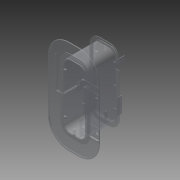
# Autodesk Inventor part: coil_former_lv_new
Saved by Autodesk Inventor 2014 SP1 (Build 180222100, 222)
## iProperties
Created: 2016-09-07
Part Number: coil_former_lv_new
Material: Polycarbonate, Clear
Document SubType Name: Modeling
Designer: tguillod
Density: 1.2 g/cm^3
Appearance: Polycarbonate - Clear
Author: tguillod
Autodesk Inventor part; units mm, degrees
ref_plane "YZ Plane" through (0, 0, 0) normal (1, 0, 0) x (0, 1, 0)
ref_plane "XZ Plane" through (0, 0, 0) normal (0, 1, 0) x (-1, 0, 0)
ref_plane "XY Plane" through (0, 0, 0) normal (0, 0, 1) x (1, 0, 0)
sketch "Sketch1" plane through (0, 0, 0) normal (0, 0, 1) x (1, 0, 0)
  line L0 (0, 0) -> (28, 0)
  line L1 (28, 0) -> (28, 1)
  line L2 (28, 1) -> (1, 1)
  line L3 (1, 1) -> (1, 3)
  line L4 (1, 3) -> (8, 3)
  line L5 (8, 3) -> (8, 4)
  line L6 (8, 4) -> (1, 4)
  line L7 (1, 4) -> (1, 55.5)
  line L8 (1, 55.5) -> (8, 55.5)
  line L9 (8, 55.5) -> (8, 56.5)
  line L10 (8, 56.5) -> (1, 56.5)
  line L11 (1, 56.5) -> (1, 59.5)
  line L12 (1, 59.5) -> (0, 59.5)
  line L13 (0, 59.5) -> (0, 0)
  line L14 (1, 58.5) -> (2, 58.5)
  line L15 (2, 58.5) -> (2, 57.5)
  line L16 (2, 57.5) -> (1, 57.5)
  line L17 (1, 57.5) -> (1, 58.5)
  line L18 (27, 1) -> (26, 1)
  line L19 (26, 1) -> (26, 2)
  line L20 (26, 2) -> (27, 2)
  line L21 (27, 2) -> (27, 1)
  dimension "d0" = 1
  dimension "d1" = 1
  dimension "d2" = 1
  dimension "d3" = 1
  dimension "d7" = 7
  dimension "d8" = 28
  dimension "d11" = 3
  dimension "d12" = 3
  dimension "d13" = 59.5
  dimension "d14" = 1
  dimension "d15" = 1
  dimension "d16" = 1
  dimension "d17" = 1
  dimension "d18" = 1
  dimension "d19" = 1
  dimension "d25" = 51.5
  constraints: 44 end point, 16 parallel, 3 collinear, 3 horizontal, 3 perpendicular, 2 point on line
  measures "d0" distance of L0.end L1.end
  measures "d1" distance of L4.end L5.end
  measures "d2" distance of L8.end L9.end
  measures "d3" distance of L11.end L12.end
  measures "d7" distance of L7.end L8.end
  measures "d8" distance of L0.start L0.end
  measures "d11" distance between parallel lines of L10 L12
  measures "d12" distance between parallel lines of L4 L0
  measures "d13" distance of L12.end L0.start
  measures "d14" distance of L18.end L19.end
  measures "d15" distance between parallel lines of L1 L21
  measures "d16" distance of L19.end L20.end
  measures "d17" distance of L15.end L16.end
  measures "d18" distance of L14.end L15.end
  measures "d19" distance between parallel lines of L12 L14
  measures "d25" distance between parallel lines of L6 L8
sketch "Sketch2" plane through (0, 0, 0) normal (0, 1, 0) x (-1, 0, 0)
  line L0 (0, 0) -> (0, 46.75)
  line L1 (10, 56.75) -> (18.5, 56.75)
  arc A0 (10, 56.75) -> (0, 46.75) centre (10, 46.75) ccw
  point P0 (0, 56.75)
  dimension "d20" = 56.75
  dimension "d21" = 18.5
  dimension "d22" = 10
  constraints: 4 end point, 2 point on circle, 2 point on line, 2 tangent, 1 centre point, 1 perpendicular, 1 vertical
  measures "d20" distance of L0.start point (0, 56.75)
  measures "d21" distance of point (0, 56.75) L1.end
  measures "d22" radius of A0
sweep "Sweep2" add profiles "Sketch1" path "Sketch2" path curves L0 A0 L1
sketch "Sketch3" plane through (0, 0, 0) normal (-1, 0, 0) x (0, 0, 1)
  line L0 (0, 59.5) -> (0, 0) projected
  line L1 (0, 0) -> (46.75, 0) projected
  line L2 (0, 59.5) -> (46.75, 59.5) projected
  line L3 (38, 59.5) -> (35, 59.5)
  line L4 (35, 59.5) -> (35, 56.5)
  line L5 (35, 56.5) -> (38, 56.5)
  line L6 (38, 56.5) -> (38, 59.5)
  line L7 (35, 0) -> (38, 0)
  line L8 (38, 0) -> (38, 3)
  line L9 (38, 3) -> (35, 3)
  line L10 (35, 3) -> (35, 0)
  dimension "d26" = 3
  dimension "d27" = 3
  dimension "d28" = 35
  constraints: 16 end point, 4 parallel, 3 collinear, 2 horizontal, 2 perpendicular, 2 point on line
  measures "d26" distance of L3.end L4.end
  measures "d27" distance of L4.end L5.end
  measures "d28" distance between parallel lines of L4 L0
extrude "Extrusion1" add sketch "Sketch3" along normal blind 4
sketch "Sketch4" plane through (-10, 0, 56.75) normal (0, 0, -1) x (-1, 0, 0)
  line L0 (8.5, 59.5) -> (7, 59.5)
  line L1 (7, 59.5) -> (7, 56.5)
  line L2 (7, 56.5) -> (8.5, 56.5)
  line L3 (8.5, 56.5) -> (8.5, 59.5)
  line L4 (8.5, 0) -> (7, 0)
  line L5 (7, 0) -> (7, 3)
  line L6 (7, 3) -> (8.5, 3)
  line L7 (8.5, 3) -> (8.5, 0)
  point P0 (-10, 0)
  dimension "d31" = 1.5
  dimension "d32" = 3
  constraints: 16 end point, 4 parallel, 2 collinear, 2 horizontal, 2 perpendicular
  measures "d31" distance of L5.end L6.end
  measures "d32" distance of L4.end L5.end
extrude "Extrusion2" add sketch "Sketch4" along normal blind 10
mirror "Mirror1" about plane through (-18.5, 58, 58.25) normal (-1, 0, 0)
mirror "Mirror2" about plane through (-38.5, 58, 0) normal (0, 0, -1)
sketch "Sketch5" plane through (1, 56.5, 0) normal (0, 1, 0) x (1, 0, 0)
  line L0 (7, 0) -> (0, 0) projected
  line L1 (0, 0) -> (0, -46.75) projected
  line L2 (0, -30) -> (10, -30)
  line L3 (10, -30) -> (10, -40)
  line L4 (10, -40) -> (0, -40)
  line L5 (0, -40) -> (0, -30)
  point P0 (-1, 0)
  dimension "d35" = 30
  dimension "d36" = 10
  dimension "d37" = 10
  constraints: 8 end point, 2 parallel, 1 horizontal, 1 perpendicular, 1 point on line
  measures "d35" distance between parallel lines of L0 L2
  measures "d36" distance of L3.end L4.end
  measures "d37" distance of L2.end L3.end
extrude "Extrusion3" cut sketch "Sketch5" along normal through all both and the other way through all
sketch "Sketch7" plane through (-27, 0, 84.75) normal (0, -1, 0) x (1, 0, 0)
  line L0 (55, -131.5) -> (55, -38) projected
  line L1 (48, -114.25) -> (53, -114.25)
  line L2 (53, -114.25) -> (53, -118.25)
  line L3 (53, -118.25) -> (48, -118.25)
  line L4 (48, -118.25) -> (48, -114.25)
  point P0 (27, -84.75)
  dimension "d45" = 29.5
  dimension "d46" = 2
  dimension "d47" = 5
  dimension "d48" = 4
  constraints: 8 end point, 2 parallel, 1 horizontal, 1 perpendicular
  measures "d45" distance from line of L1 point (27, -84.75)
  measures "d46" distance between parallel lines of L0 L2
  measures "d47" distance of L2.end L3.end
  measures "d48" distance of L1.end L2.end
extrude "Extrusion5" cut sketch "Sketch7" against normal blind 10
fillet "Fillet1" radius 3 2 edges at (11, 0.5, 30) (11, 0.5, 40)
sketch "Sketch8" plane through (-27, 0, 84.75) normal (0, -1, 0) x (1, 0, 0)
  line L0 (48, -114.25) -> (53, -114.25) projected
  line L1 (53, -118.25) -> (48, -118.25) projected
  line L2 (27, -49.75) -> (27, -119.75) projected
  line L3 (55, -131.5) -> (55, -38) projected
  line L4 (30, -106.25) -> (55, -106.25)
  line L5 (55, -106.25) -> (55, -107.25)
  line L6 (55, -107.25) -> (30, -107.25)
  line L7 (30, -107.25) -> (30, -106.25)
  line L8 (55, -125.25) -> (30, -125.25)
  line L9 (30, -125.25) -> (30, -126.25)
  line L10 (30, -126.25) -> (55, -126.25)
  line L11 (55, -126.25) -> (55, -125.25)
  point P0 (27, -84.75)
  dimension "d52" = 3
  dimension "d53" = 1
  dimension "d54" = 1
  dimension "d55" = 7
  dimension "d56" = 7
  constraints: 16 end point, 3 equal length, 2 horizontal, 2 perpendicular, 2 point on line, 1 collinear
  measures "d52" distance between parallel lines of L2 L7
  measures "d53" distance of L6.end L4.start
  measures "d54" distance of L8.end L9.end
  measures "d55" distance between parallel lines of L6 L0
  measures "d56" distance between parallel lines of L1 L8
extrude "Extrusion6" add sketch "Sketch8" along normal blind 3
sketch "Sketch9" plane through (28, 0, -41.5) normal (0, 0, -1) x (-1, 0, 0)
  line L0 (25, 0) -> (25, -3) projected
  line L1 (0, -3) -> (25, -3)
  line L2 (25, -3) -> (25, -2)
  line L3 (25, -2) -> (0, -2)
  line L4 (0, -2) -> (0, -3)
  point P0 (28, 0)
  dimension "d59" = 1
  constraints: 8 end point, 2 parallel, 1 horizontal, 1 perpendicular, 1 point on line
  measures "d59" distance of L3.end L1.start
extrude "Extrusion7" add sketch "Sketch9" along normal blind 1
sketch "Sketch10" plane through (3, 0, -21.5) normal (0, 0, 1) x (1, 0, 0)
  line L0 (25, 0) -> (25, -3) projected
  line L1 (0, -3) -> (25, -3)
  line L2 (25, -3) -> (25, -2)
  line L3 (25, -2) -> (0, -2)
  line L4 (0, -2) -> (0, -3)
  point P0 (-3, 0)
  dimension "d62" = 1
  constraints: 8 end point, 2 parallel, 1 horizontal, 1 perpendicular, 1 point on line
  measures "d62" distance of L1.end L2.end
extrude "Extrusion8" add sketch "Sketch10" along normal blind 1
sketch "Sketch11" plane through (-27, 0, 84.75) normal (0, -1, 0) x (1, 0, 0)
  line L0 (27, -49.75) -> (27, -119.75) projected
  line L1 (55, -126.25) -> (30, -126.25) projected
  line L2 (30, -106.25) -> (55, -106.25) projected
  line L3 (27, -102.25) -> (28, -102.25)
  line L4 (28, -102.25) -> (28, -130.25)
  line L5 (28, -130.25) -> (27, -130.25)
  line L6 (27, -130.25) -> (27, -102.25)
  point P0 (27, -84.75)
  dimension "d65" = 1
  dimension "d67" = 4
  dimension "d68" = 4
  constraints: 8 end point, 2 parallel, 1 collinear, 1 horizontal, 1 perpendicular
  measures "d65" distance of L3.start L3.end
  measures "d67" distance between parallel lines of L3 L2
  measures "d68" distance between parallel lines of L1 L5
extrude "Extrusion9" add sketch "Sketch11" along normal blind 7
sketch "Sketch12" plane through (-27, -7, 84.75) normal (0, -1, 0) x (1, 0, 0)
  line L0 (27, -102.25) -> (28, -102.25)
  line L1 (28, -102.25) -> (28, -130.25)
  line L2 (28, -130.25) -> (27, -130.25)
  line L3 (27, -130.25) -> (27, -102.25)
  point P0 (27, -84.75)
  constraints: 8 end point, 2 parallel, 1 horizontal, 1 perpendicular
extrude "Extrusion10" add sketch "Sketch12" along normal blind 1
sketch "Sketch13" plane through (-27, 0, 84.75) normal (0, -1, 0) x (1, 0, 0)
  line L0 (55, -106.25) -> (55, -38) projected
  line L1 (28, -44.75) -> (55, -44.75)
  line L2 (55, -44.75) -> (55, -43.75)
  line L3 (55, -43.75) -> (28, -43.75)
  line L4 (28, -43.75) -> (28, -44.75)
  line L5 (28, -54.75) -> (55, -54.75)
  line L6 (55, -54.75) -> (55, -55.75)
  line L7 (55, -55.75) -> (28, -55.75)
  line L8 (28, -55.75) -> (28, -54.75)
  point P0 (27, -84.75)
  dimension "d79" = 1
  dimension "d80" = 1
  constraints: 16 end point, 4 parallel, 2 horizontal, 2 perpendicular, 2 point on line
  measures "d79" distance between parallel lines of L1 L3
  measures "d80" distance between parallel lines of L7 L5
extrude "Extrusion11" add sketch "Sketch13" along normal blind 1
sketch "Sketch15" plane through (-27, 0, 84.75) normal (0, -1, 0) x (1, 0, 0)
  line L0 (-10, -119.75) -> (-10, -49.75) construction
  line L1 (-20, -83.25) -> (-9, -83.25)
  line L2 (-9, -83.25) -> (-9, -84.25)
  line L3 (-9, -84.25) -> (-20, -84.25)
  line L4 (-20, -84.25) -> (-20, -83.25)
  line L5 (-22, -85.25) -> (-9, -85.25)
  line L6 (-9, -85.25) -> (-9, -86.25)
  line L7 (-9, -86.25) -> (-22, -86.25)
  line L8 (-22, -86.25) -> (-22, -85.25)
  line L9 (-23, -28.25) -> (-22, -28.25)
  line L10 (-22, -28.25) -> (-22, -86.25)
  line L11 (-22, -86.25) -> (-23, -86.25)
  line L12 (-23, -86.25) -> (-23, -28.25)
  line L13 (-21, -28.25) -> (-20, -28.25)
  line L14 (-20, -28.25) -> (-20, -84.25)
  line L15 (-20, -84.25) -> (-21, -84.25)
  line L16 (-21, -84.25) -> (-21, -28.25)
  point P0 (27, -84.75)
  point P1 (-10, -84.75)
  dimension "d88" = 0.5
  dimension "d89" = 0.5
  dimension "d90" = 1
  dimension "d91" = 1
  dimension "d92" = 1
  dimension "d93" = 1
  dimension "d94" = 1
  dimension "d95" = 1
  dimension "d96" = 10
  dimension "d103" = 58
  constraints: 32 end point, 8 parallel, 6 collinear, 4 horizontal, 4 perpendicular, 1 midpoint
  measures "d88" distance from line of point (-10, -84.75) L3
  measures "d89" distance from line of point (-10, -84.75) L5
  measures "d90" distance between parallel lines of L2 L0
  measures "d91" distance of L1.end L2.end
  measures "d92" distance of L5.end L6.end
  measures "d93" distance of L9.start L9.end
  measures "d94" distance of L13.start L13.end
  measures "d95" distance between parallel lines of L10 L16
  measures "d96" distance between parallel lines of L14 L0
  measures "d103" distance of L11.end L9.start
extrude "Extrusion12" add sketch "Sketch15" along normal blind 1
sketch "Sketch17" plane through (-27, 0, 84.75) normal (0, 1, 0) x (1, 0, 0)
  line L0 (-10, 84.25) -> (-10, 83.25) projected
  line L1 (-10, 83.25) -> (-9, 83.25) projected
  line L2 (-9, 83.25) -> (-9, 84.25) projected
  line L3 (-9, 84.25) -> (-10, 84.25) projected
  line L4 (-9, 86.25) -> (-10, 86.25)
  line L5 (-10, 86.25) -> (-10, 85.25)
  line L6 (-10, 85.25) -> (-9, 85.25)
  line L7 (-9, 85.25) -> (-9, 86.25)
  line L8 (-10, 84.25) -> (-9, 84.25)
  line L9 (-9, 84.25) -> (-9, 83.25)
  line L10 (-9, 83.25) -> (-10, 83.25)
  line L11 (-10, 83.25) -> (-10, 84.25)
  point P0 (27, 84.75)
  constraints: 16 end point, 4 parallel, 2 horizontal, 2 perpendicular
extrude "Extrusion14" add sketch "Sketch17" along normal blind 29.75
fillet "Fillet4" radius 1 12 edges at (-18.5, 0, -84.75) (-53.8701, 0, -73.6201) (-65, 0, 0) (-53.8701, 0, 73.6201) (-18.5, 0, 84.75) (16.8701, 0, 73.6201) (28, 0, 43.875) (28, 0, -44.125) (16.8701, 0, -73.6201) (28, 0, 35) (28, 0, 3.75) (28, 0, -31.5)
fillet "Fillet5" radius 1 6 edges at (27.7071, 0.2929, -41.5) (15, 0, -41.5) (15.5, -2, -41.5) (27.7071, 0.2929, -21.5) (15, 0, -21.5) (15.5, -2, -21.5)
sketch "Sketch20" plane through (1, 0, 30) normal (0, -1, 0) x (1, 0, 0)
  line L0 (0, 0) -> (0, 10) projected
  line L1 (-1, 8) -> (-1, 16.75) projected
  line L2 (-1, 12) -> (0, 12)
  line L3 (0, 12) -> (0, -2)
  line L4 (0, -2) -> (-1, -2)
  line L5 (-1, -2) -> (-1, 12)
  line L6 (0, 10) -> (27, 10) projected
  line L7 (27, 0) -> (0, 0) projected
  point P0 (-1, -30)
  dimension "d111" = 2
  dimension "d112" = 2
  constraints: 8 end point, 2 parallel, 1 collinear, 1 horizontal, 1 perpendicular, 1 point on line
  measures "d111" distance between parallel lines of L2 L6
  measures "d112" distance between parallel lines of L4 L7
extrude "Extrusion16" add sketch "Sketch20" along normal blind 13
sketch "Sketch21" plane through (-27, 59.5, 57.75) normal (0, 1, 0) x (1, 0, 0)
  line L0 (27, 75.25) -> (27, 103.25) projected
  line L1 (27, 103.25) -> (28, 103.25) projected
  line L2 (28, 103.25) -> (28, 75.25) projected
  line L3 (28, 75.25) -> (27, 75.25) projected
  line L4 (28, 103.25) -> (27, 103.25)
  line L5 (27, 103.25) -> (27, 75.25)
  line L6 (27, 75.25) -> (28, 75.25)
  line L7 (28, 75.25) -> (28, 103.25)
  point P0 (27, 57.75)
  constraints: 8 end point, 2 parallel, 1 horizontal, 1 perpendicular
extrude "Extrusion17" add sketch "Sketch21" along normal blind 8
sketch "Sketch22" plane through (0, 59.5, 46.75) normal (0, 1, 0) x (1, 0, 0)
  line L0 (0, 4.75) -> (0, 18.75) projected
  line L1 (0, 18.75) -> (1, 18.75) projected
  line L2 (1, 18.75) -> (1, 4.75) projected
  line L3 (1, 4.75) -> (0, 4.75) projected
  line L4 (0, 18.75) -> (1, 18.75)
  line L5 (1, 18.75) -> (1, 4.75)
  line L6 (1, 4.75) -> (0, 4.75)
  line L7 (0, 4.75) -> (0, 18.75)
  point P0 (0, 46.75)
  constraints: 8 end point, 2 parallel, 1 horizontal, 1 perpendicular
extrude "Extrusion18" add sketch "Sketch22" along normal blind 13
sketch "Sketch23" plane through (0, 0, 46.75) normal (-1, 0, 0) x (0, 0, 1)
  line L0 (-64.25, 59.5) -> (-18.75, 59.5) projected
  line L1 (-18.75, 0) -> (-64.25, 0) projected
  line L2 (-11.75, 56.5) -> (-11.75, 59.5) projected
  line L3 (-81.75, 56.5) -> (-81.75, 59.5) projected
  line L4 (-48.25, 0) -> (-45.25, 0)
  line L5 (-45.25, 0) -> (-45.25, 3)
  line L6 (-45.25, 3) -> (-48.25, 3)
  line L7 (-48.25, 3) -> (-48.25, 0)
  line L8 (-48.25, 59.5) -> (-45.25, 59.5)
  line L9 (-45.25, 59.5) -> (-45.25, 56.5)
  line L10 (-45.25, 56.5) -> (-48.25, 56.5)
  line L11 (-48.25, 56.5) -> (-48.25, 59.5)
  point P0 (-46.75, 0)
  dimension "d119" = 3
  dimension "d120" = 3
  dimension "d121" = 3
  dimension "d122" = 3
  dimension "d123" = 33.5
  dimension "d124" = 33.5
  constraints: 16 end point, 4 parallel, 2 horizontal, 2 perpendicular, 2 point on line, 1 collinear
  measures "d119" distance of L5.end L6.end
  measures "d120" distance of L4.end L5.end
  measures "d121" distance of L9.end L10.end
  measures "d122" distance of L8.end L9.end
  measures "d123" distance between parallel lines of L2 L9
  measures "d124" distance between parallel lines of L3 L11
extrude "Extrusion19" add sketch "Sketch23" along normal blind 4
body "Solid2"
